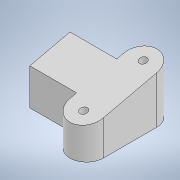
# Autodesk Inventor part: Проставка для двигателя
Saved by Autodesk Inventor 2020 (Build 240168000, 168)
## iProperties
Created: 2021-06-02
Part Number: Проставка для двигателя
Material: Типовые
Document SubType Name: Modeling
Designer: Антон
Density: 1 g/cm^3
Appearance: По умолчанию
Author: Антон
Autodesk Inventor part; units mm, degrees
ref_plane "YZ Plane" through (0, 0, 0) normal (1, 0, 0) x (0, 1, 0)
ref_plane "XZ Plane" through (0, 0, 0) normal (0, 1, 0) x (-1, 0, 0)
ref_plane "XY Plane" through (0, 0, 0) normal (0, 0, 1) x (1, 0, 0)
sketch "Эскиз1" plane through (0, 0, 0) normal (0, 1, 0) x (-1, 0, 0)
  line L0 (0, 0) -> (0, -16) construction
  line L1 (-5, 0) -> (-5, -16)
  line L2 (5, -16) -> (5, 0)
  arc A0 (5, 0) -> (-5, 0) centre (0, 0) ccw
  arc A1 (-5, -16) -> (5, -16) centre (0, -16) ccw
  line L3 (5, -14) -> (19, -14)
  line L4 (19, -14) -> (19, -2)
  line L5 (19, -2) -> (5, -2)
  line L6 (5, -2) -> (5, -14)
  circle A2 centre (0, -16.9) radius 1.1
  circle A3 centre (0, 0.9) radius 1.1
  line L7 (0, -16.9) -> (0, 0.9)
  point P0 (0, -8)
  point P1 (5, -8)
  point P2 (5, -2)
  point P3 (5, -14)
  point P4 (0, -8)
  dimension "d0" = 16
  dimension "d1" = 5
  dimension "d3" = 24
  dimension "d4" = 12
  dimension "d8" = 17.8
  dimension "d9" = 2.2
  constraints: 18 end point, 4 centre point, 4 midpoint, 4 point on circle, 4 tangent, 3 coincident, 3 parallel, 1 collinear, 1 equal radius, 1 horizontal, 1 perpendicular, 1 vertical
  measures "d0" distance of L0.start L0.end
  measures "d1" radius of A1
  measures "d3" distance between parallel lines of L1 L4
  measures "d4" distance of L3.end L4.end
  measures "d8" distance of L7.start L7.end
  measures "d9" diameter of A2
extrude "Выдавливание1" add sketch "Эскиз1" along normal blind 15.3
sketch "Эскиз2" plane through (5, 0, 0) normal (1, 0, 0) x (0, 0, -1)
  line L0 (21, 15.3) -> (16, 15.3) projected
  line L1 (21, 15.3) -> (-5, 9.3)
  line L2 (-5, 0) -> (-5, 15.3) projected
  line L3 (-5, 9.3) -> (20.5284, 9.3)
  line L4 (20.5284, 9.3) -> (21, 9.3)
  line L5 (21, 15.3) -> (21, 9.3)
  line L6 (21, 0) -> (21, 15.3) projected
  line L7 (0, 15.3) -> (16, 15.3) projected
  line L8 (0, 15.3) -> (-5, 15.3) projected
  point P0 (0, 0)
  dimension "d10" = 6
  constraints: 8 end point, 2 point on line, 1 collinear, 1 horizontal
  measures "d10" distance of L0.start L4.end
extrude "Выдавливание2" cut sketch "Эскиз2" against normal through all contours L1 L2 L8 L7 L0
